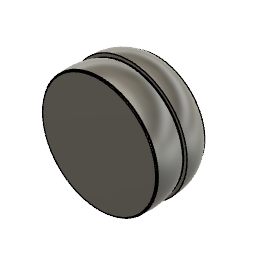
answer (Autodesk Fusion 360 design; units mm, degrees)
part number: 2026-08-05-21-59-05-398
Autodesk Fusion 360 part; units mm, degrees
sketch "Sketch1" plane through (0, 0, 0) normal (0, 1, 0) x (1, 0, 0)
  line L0 (0, 0) -> (-35, 0)
  line L1 (0, 0) -> (0, -20)
  line L2 (0, -20) -> (-42, -20)
  arc A0 (-35, 0) -> (-42, -20) centre (-17.1273, -17.4804) ccw
  dimension "d1" = 35
  dimension "d2" = 20
  dimension "d3" = 42
  dimension "d4" = 25
  constraint coincident L0.start L1.start
  constraint horizontal L0
  constraint perpendicular L0 L1
  constraint perpendicular L1 L2
  measures "d1" distance of L0.start L0.end
  measures "d2" distance of L0.start L1.end
  measures "d3" distance of L1.end L2.end
  measures "d4" radius of A0
revolve "Revolve1" add sketch "Sketch1" angle 360 about axis through (0, 0, 0) along (0, 0, 1)
sketch "Sketch2" plane through (0, 0, 20) normal (0, 0, 1) x (1, 0, 0)
  circle A0 centre (0, 0) radius 42
  circle A1 centre (0, 0) radius 39.5
  dimension "d6" = 79
  constraint concentric A0 A1
  measures "d6" diameter of A1
extrude "Extrude1" add sketch "Sketch2" along normal blind 1 contours A1
sketch "Sketch4" plane through (0, 0, 21) normal (0, 0, 1) x (1, 0, 0)
  circle A0 centre (0, 0) radius 39.5
  constraint coincident A0.centre origin
sketch "Sketch5" plane through (0, 0, 0) normal (0, 1, 0) x (1, 0, 0)
  line L0 (0, -21) -> (0, -41)
  line L1 (0, -41) -> (-42, -41)
  line L2 (0, -21) -> (-40, -21)
  arc A0 (-40, -21) -> (-42, -41) centre (-5.5677, -34.5432) ccw
  point P0 (0, -21)
  dimension "d9" = 20
  dimension "d10" = 42
  dimension "d11" = 40
  dimension "d12" = 37
  constraint vertical L0
  constraint perpendicular L0 L1
  constraint perpendicular L0 L2
  constraint coincident L0 P0
  measures "d9" distance of P0 L0.end
  measures "d10" distance of L0.end L1.end
  measures "d11" distance of P0 L2.end
  measures "d12" radius of A0
revolve "Revolve2" add sketch "Sketch5" angle 360 about axis through (0, 0, 1.75) along (0, 0, 1)
sketch "Sketch6" plane through (0, 0, 41) normal (0, 0, 1) x (1, 0, 0)
  circle A0 centre (0, 0) radius 42
  circle A1 centre (0, 0) radius 41.25
  dimension "d14" = 82.5
  constraint concentric A0 A1
  measures "d14" diameter of A1
extrude "Extrude2" add sketch "Sketch6" along normal blind 1 contours A1
